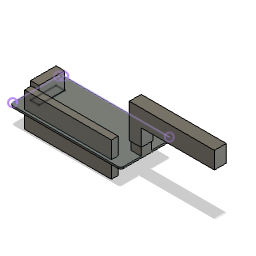
LoRa HAT (Autodesk Fusion 360 design; units mm, degrees)
Autodesk Fusion 360 part; units mm, degrees
sketch "Sketch1" plane through (0, 0, 0) normal (0, 1, 0) x (1, 0, 0)
  line L0 (1.5, 0) -> (63.5, 0)
  line L1 (65, -1.5) -> (65, -28.5)
  line L2 (63.5, -30) -> (1.5, -30)
  line L3 (0, -28.5) -> (0, -1.5)
  arc A0 (1.5, 0) -> (0, -1.5) centre (1.5, -1.5) ccw
  arc A1 (65, -1.5) -> (63.5, 0) centre (63.5, -1.5) ccw
  arc A2 (63.5, -30) -> (65, -28.5) centre (63.5, -28.5) ccw
  arc A3 (0, -28.5) -> (1.5, -30) centre (1.5, -28.5) ccw
  point P0 (65, 0)
  point P1 (0, -30)
  dimension "d1" = 65
  dimension "d2" = 30
  dimension "d3" = 1.5
  dimension "d4" = 1.5
  dimension "d5" = 1.5
  dimension "d6" = 1.5
  constraint horizontal L0
  constraint vertical L1
  constraint horizontal L2
  constraint vertical L3
  constraint coincident origin L0
  constraint coincident origin L3
  constraint tangent L0 A0
  constraint tangent L3 A0
  constraint coincident P0 L0
  constraint coincident P0 L1
  constraint tangent L0 A1
  constraint tangent L1 A1
  constraint tangent L1 A2
  constraint tangent L2 A2
  constraint coincident P1 L2
  constraint coincident P1 L3
  constraint tangent L2 A3
  constraint tangent L3 A3
  measures "d1" distance of origin P0
  measures "d2" distance of origin P1
  measures "d3" radius of A0
  measures "d4" radius of A1
  measures "d5" radius of A2
  measures "d6" radius of A3
extrude "Extrude6" add sketch "Sketch1" along normal blind 1 makes body 1
sketch "Sketch4" plane through (0, 1, 0) normal (0, 1, 0) x (-1, 0, 0)
  arc A0 (-1.5, 0) -> (0, 1.5) centre (-1.5, 1.5) ccw
  line L0 (0, 1.5) -> (0, 28.5)
  arc A1 (0, 28.5) -> (-1.5, 30) centre (-1.5, 28.5) ccw
  line L1 (-1.5, 30) -> (-63.5, 30)
  arc A2 (-63.5, 30) -> (-65, 28.5) centre (-63.5, 28.5) ccw
  line L2 (-65, 28.5) -> (-65, 1.5)
  arc A3 (-65, 1.5) -> (-63.5, 0) centre (-63.5, 1.5) ccw
  line L3 (-63.5, 0) -> (-1.5, 0)
  line L4 (0, 28.5) -> (-7, 28.5) construction
  line L5 (-65, 28.5) -> (-58, 28.5) construction
  line L6 (-7, 28.5) -> (-58, 28.5)
  line L7 (-58, 28.5) -> (-58, 24.5)
  line L8 (-58, 24.5) -> (-7, 24.5)
  line L9 (-7, 24.5) -> (-7, 28.5)
  dimension "d20" = 7
  dimension "d21" = 7
  dimension "d22" = 4
  dimension "d57" = 7
  dimension "d58" = 7
  constraint coincident L0.end A1.start
  constraint perpendicular L0 L4
  constraint coincident A2.end L2.start
  constraint perpendicular L2 L5
  constraint horizontal L6
  constraint vertical L7
  constraint horizontal L8
  constraint vertical L9
  measures "d20" distance of L0.end L4.end
  measures "d21" distance of A2.end L5.end
  measures "d22" distance of L4.end L8.end
  measures "d57" distance of L2 L7
  measures "d58" distance of L0 L9
extrude "Extrude7" add sketch "Sketch4" along normal blind 10 contours L6 L7 L8 L9 bodies 1
sketch "Sketch6" plane through (0, 1, 0) normal (0, 1, 0) x (-1, 0, 0)
  line L0 (-7, 24.5) -> (-58, 24.5)
  line L1 (-58, 24.5) -> (-58, 28.5)
  line L2 (-58, 28.5) -> (-7, 28.5)
  line L3 (-7, 28.5) -> (-7, 24.5)
  arc A0 (-1.5, 0) -> (0, 1.5) centre (-1.5, 1.5) ccw
  line L4 (0, 1.5) -> (0, 28.5)
  arc A1 (0, 28.5) -> (-1.5, 30) centre (-1.5, 28.5) ccw
  line L5 (-1.5, 30) -> (-63.5, 30)
  arc A2 (-63.5, 30) -> (-65, 28.5) centre (-63.5, 28.5) ccw
  line L6 (-65, 28.5) -> (-65, 1.5)
  arc A3 (-65, 1.5) -> (-63.5, 0) centre (-63.5, 1.5) ccw
  line L7 (-63.5, 0) -> (-1.5, 0)
  line L8 (-59, 12) -> (-65, 12)
  line L9 (-65, 12) -> (-65, 18)
  line L10 (-65, 18) -> (-59, 18)
  line L11 (-59, 18) -> (-59, 12)
  line L12 (-1.5, 0) -> (-63.5, 0)
  line L13 (-63.5, 30) -> (-1.5, 30)
  line L14 (-65, 1.5) -> (-65, 28.5)
  dimension "d29" = 6
  dimension "d30" = 6
  constraint horizontal L8
  constraint vertical L9
  constraint horizontal L10
  constraint vertical L11
  constraint midpoint L9 L14
  measures "d29" distance of L8.start L8.end
  measures "d30" distance of L8.start L10.end
extrude "Extrude8" add sketch "Sketch6" along normal blind 5 contours L6 L8 L9 L10 L11 L14 bodies 1
sketch "Sketch7" plane through (0, 1, 0) normal (0, 1, 0) x (-1, 0, 0)
  line L0 (-65, 18) -> (-59, 18)
  line L1 (-59, 18) -> (-59, 12)
  line L2 (-59, 12) -> (-65, 12)
  line L3 (-65, 12) -> (-65, 1.5)
  arc A0 (-65, 1.5) -> (-63.5, 0) centre (-63.5, 1.5) ccw
  line L4 (-63.5, 0) -> (-1.5, 0)
  arc A1 (-1.5, 0) -> (0, 1.5) centre (-1.5, 1.5) ccw
  line L5 (0, 1.5) -> (0, 28.5)
  arc A2 (0, 28.5) -> (-1.5, 30) centre (-1.5, 28.5) ccw
  line L6 (-1.5, 30) -> (-63.5, 30)
  arc A3 (-63.5, 30) -> (-65, 28.5) centre (-63.5, 28.5) ccw
  line L7 (-65, 28.5) -> (-65, 18)
  line L8 (-7, 24.5) -> (-58, 24.5)
  line L9 (-58, 24.5) -> (-58, 28.5)
  line L10 (-58, 28.5) -> (-7, 28.5)
  line L11 (-7, 28.5) -> (-7, 24.5)
  line L12 (-4, 7) -> (-9, 7)
  line L13 (-9, 7) -> (-9, 22)
  line L14 (-9, 22) -> (-4, 22)
  line L15 (-4, 22) -> (-4, 7)
  line L16 (0, 28.5) -> (0, 1.5)
  line L17 (-1.5, 0) -> (-63.5, 0)
  dimension "d38" = 5
  dimension "d39" = 15
  dimension "d40" = 4
  dimension "d41" = 7
  constraint horizontal L12
  constraint vertical L13
  constraint horizontal L14
  constraint vertical L15
  measures "d38" distance of L12.start L12.end
  measures "d39" distance of L12.start L14.end
  measures "d40" distance of L15 L16
  measures "d41" distance of L12 L17
extrude "Extrude9" add sketch "Sketch7" along normal blind 10 contours L12 L13 L14 L15 bodies 1
sketch "Sketch8" plane through (0, 6, 0) normal (0, 1, 0) x (-1, 0, 0)
  line L0 (-59, 12) -> (-59, 18)
  line L1 (-59, 18) -> (-65, 18)
  line L2 (-65, 18) -> (-65, 12)
  line L3 (-65, 12) -> (-59, 12)
  line L4 (-58.5, 11.5) -> (-65.5, 11.5)
  line L5 (-65.5, 11.5) -> (-65.5, 18.5)
  line L6 (-65.5, 18.5) -> (-58.5, 18.5)
  line L7 (-58.5, 18.5) -> (-58.5, 11.5)
  line L8 (-58.5, 11.5) -> (-65.5, 18.5) construction
  line L9 (-65.5, 11.5) -> (-58.5, 18.5) construction
  point P0 (-62, 15)
  point P1 (-62, 15)
  dimension "d46" = 3
  dimension "d47" = 3
  dimension "d48" = 7
  dimension "d49" = 7
  constraint horizontal L4
  constraint perpendicular L4 L5
  constraint parallel L4 L6
  constraint parallel L5 L7
  constraint coincident L8 P1
  constraint coincident L9 P1
  constraint coincident P1 P0
  measures "d46" distance of L2 P1
  measures "d47" distance of L3 P1
  measures "d48" distance of L5.end L6.end
  measures "d49" distance of L4.end L5.end
extrude "Extrude1" add sketch "Sketch8" along normal blind 20 separate body contours L0 L1 L2 L3 | L4 L5 L6 L7 makes body 2 in component "Antenna"
sketch "Sketch1 (2)" plane through (65.5, 0, 0) normal (1, 0, 0) x (0, 0, -1) in component "Antenna"
  line L0 (-18.5, 6) -> (-11.5, 6)
  line L1 (-11.5, 6) -> (-11.5, 26)
  line L2 (-11.5, 26) -> (-18.5, 26)
  line L3 (-18.5, 26) -> (-18.5, 6)
  line L4 (-18.5, 26) -> (-11.5, 26)
  line L5 (-11.5, 26) -> (-11.5, 16)
  line L6 (-11.5, 16) -> (-18.5, 16)
  line L7 (-18.5, 16) -> (-18.5, 26)
  dimension "d52" = 10
  constraint horizontal L4
  constraint vertical L5
  constraint horizontal L6
  constraint vertical L7
  constraint coincident L2.end L3.start
  measures "d52" distance of L2.end L6.end
extrude "Extrude2" add sketch "Sketch1 (2)" along normal blind 43 contours L1 L2 L3 L4 L5 L6 L7 bodies 2 in component "Antenna"
sketch "Sketch10" plane through (0, 0, 0) normal (0, -1, 0) x (1, 0, 0)
  arc A0 (0, 1.5) -> (1.5, 0) centre (1.5, 1.5) ccw
  line L0 (1.5, 0) -> (63.5, 0)
  arc A1 (63.5, 0) -> (65, 1.5) centre (63.5, 1.5) ccw
  line L1 (65, 1.5) -> (65, 28.5)
  arc A2 (65, 28.5) -> (63.5, 30) centre (63.5, 28.5) ccw
  line L2 (63.5, 30) -> (1.5, 30)
  arc A3 (1.5, 30) -> (0, 28.5) centre (1.5, 28.5) ccw
  line L3 (0, 28.5) -> (0, 1.5)
  line L4 (7, 24.5) -> (58, 24.5) construction
  line L5 (58, 24.5) -> (58, 28.5) construction
  line L6 (58, 28.5) -> (7, 28.5) construction
  line L7 (7, 28.5) -> (7, 24.5) construction
  line L8 (7, 24.5) -> (58, 24.5)
  line L9 (58, 24.5) -> (58, 28.5)
  line L10 (58, 28.5) -> (7, 28.5)
  line L11 (7, 28.5) -> (7, 24.5)
  constraint horizontal L4
  constraint vertical L5
  constraint horizontal L6
  constraint vertical L7
  constraint horizontal L8
  constraint vertical L9
  constraint horizontal L10
  constraint vertical L11
extrude "Extrude10" add sketch "Sketch10" along normal blind 9 contours L8 L9 L10 L11 bodies 1
component "Antenna" placed x (1, 0, 0) y (0, 1, 0) z (0, 0, 1) at (0, 0, 0)
